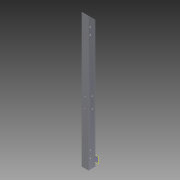
# Autodesk Inventor part: Square Tube
Saved by Autodesk Inventor 2013 (Build 170138000, 138)
## iProperties
Created: 2013-01-18
Part Number: Square Tube
Material: Aluminum 6061
Document SubType Name: Modeling
Designer: actoennies
Density: 2.71 g/cm^3
Mass: 190.087 g
Surface Area: 893.355 cm^2
Volume: 70.1426 cm^3
Author: actoennies
Autodesk Inventor part; units mm, degrees
ref_plane "YZ Plane" through (0, 0, 0) normal (1, 0, 0) x (0, 1, 0)
ref_plane "XZ Plane" through (0, 0, 0) normal (0, 1, 0) x (-1, 0, 0)
ref_plane "XY Plane" through (0, 0, 0) normal (0, 0, 1) x (1, 0, 0)
sketch "Sketch1" plane through (0, 0, 0) normal (0, 1, 0) x (-1, 0, 0)
  line L0 (0, 0) -> (-25.4, 0)
  line L1 (-25.4, 0) -> (-25.4, 25.4)
  line L2 (-25.4, 25.4) -> (0, 25.4)
  line L3 (0, 25.4) -> (0, 0)
  line L4 (-1.5875, 23.8125) -> (-23.8125, 23.8125)
  line L5 (-23.8125, 23.8125) -> (-23.8125, 1.5875)
  line L6 (-23.8125, 1.5875) -> (-1.5875, 1.5875)
  line L7 (-1.5875, 1.5875) -> (-1.5875, 23.8125)
  dimension "d0" = 25.4
  dimension "d2" = 25.4
  dimension "d3" = 22.225
  constraints: 16 end point, 4 parallel, 2 perpendicular, 1 horizontal, 3 other
  measures "d0" distance of L1.end L2.end
  measures "d2" distance of L2.end L0.start
  measures "d3" distance of L4.start L4.end
extrude "Extrusion1" add sketch "Sketch1" along normal blind 495.3
sketch "Sketch2" plane through (25.4, 0, 25.4) normal (1, 0, 0) x (0, 0, -1)
  line L0 (25.4, 0) -> (25.4, 495.3) projected
  line L1 (0, 495.3) -> (25.4, 495.3) projected
  line L2 (0, 495.3) -> (25.4, 469.9)
  point P0 (25.4, 25.4)
  dimension "d7" = 45
  constraints: 2 end point, 2 point on line
  measures "d7" angle of L1 L2
sketch "Sketch3" plane through (0, 0, 25.4) normal (-1, 0, 0) x (0, 0, 1)
  line L0 (0, 0) -> (0, 495.3) projected
  circle A0 centre (-6.35, 457.2) radius 3.3782
  circle A1 centre (-6.35, 431.8) radius 3.3782
  circle A2 centre (-6.35, 38.1) radius 3.3782
  circle A3 centre (-6.35, 63.5) radius 3.3782
  point P0 (-25.4, 0)
  dimension "d10" = 6.7564
  dimension "d11" = 6.7564
  dimension "d12" = 38.1
  dimension "d13" = 6.35
  dimension "d14" = 6.35
  dimension "d15" = 63.5
  dimension "d16" = 6.7564
  dimension "d17" = 6.7564
  dimension "d18" = 63.5
  dimension "d19" = 38.1
  dimension "d20" = 6.35
  dimension "d21" = 6.35
  constraints: 4 centre point
  measures "d10" diameter of A0
  measures "d11" diameter of A1
  measures "d12" vertical distance of L0.end A0.centre
  measures "d13" distance from line of L0 A0.centre
  measures "d14" distance from line of L0 A1.centre
  measures "d15" vertical distance of L0.end A1.centre
  measures "d16" diameter of A2
  measures "d17" diameter of A3
  measures "d18" vertical distance of L0.start A3.centre
  measures "d19" vertical distance of L0.start A2.centre
  measures "d20" distance from line of L0 A3.centre
  measures "d21" distance from line of L0 A2.centre
extrude "Extrusion3" cut sketch "Sketch3" against normal blind 25.4
ref_plane "Work Plane1" through (25.4, 25.4, 0) normal (0, 0, -1) x (-1, 0, 0)
sketch "Sketch4" plane through (25.4, 25.4, 0) normal (0, 0, -1) x (-1, 0, 0)
  circle A0 centre (12.6566, 207.0968) radius 3.3782 projected
  circle A1 centre (12.6566, 168.9968) radius 3.3782 projected
  point P0 (25.4, -25.4)
extrude "Extrusion4" cut sketch "Sketch4" against normal blind 25.4
sketch "Sketch5" plane through (25.4, 0, 25.4) normal (1, 0, 0) x (0, 0, -1)
  circle A0 centre (14.0716, 191.2218) radius 3.3782 projected
  circle A1 centre (14.0716, 232.4968) radius 3.3782 projected
  point P0 (25.4, 0)
extrude "Extrusion5" cut sketch "Sketch5" against normal blind 25.4
extrude "Extrusion6" cut sketch "Sketch2" against normal blind 25.4
body "Solid1"
